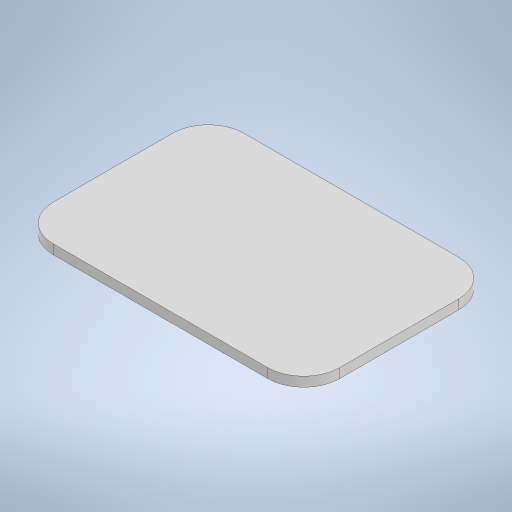
# Autodesk Inventor part: bottom ecoflex layer
Saved by Autodesk Inventor 2024.2 (Build 282272000, 272)
## iProperties
Created: 2025-02-11
Part Number: bottom ecoflex layer
Material: Generic
Document SubType Name: Modeling
Designer: Tom
Density: 1 g/cm^3
Appearance: Default
Author: Tom
Autodesk Inventor part; units mm, degrees
ref_plane "YZ Plane" through (0, 0, 0) normal (1, 0, 0) x (0, 1, 0)
ref_plane "XZ Plane" through (0, 0, 0) normal (0, 1, 0) x (-1, 0, 0)
ref_plane "XY Plane" through (0, 0, 0) normal (0, 0, 1) x (1, 0, 0)
sketch "Sketch1" plane through (0, 0, 0) normal (0, 1, 0) x (-1, 0, 0)
  line L0 (9.525, 0) -> (66.675, 0)
  line L1 (76.2, -9.525) -> (76.2, -41.275)
  line L2 (66.675, -50.8) -> (9.525, -50.8)
  line L3 (0, -41.275) -> (0, -9.525)
  arc A0 (76.2, -9.525) -> (66.675, 0) centre (66.675, -9.525) ccw
  arc A1 (66.675, -50.8) -> (76.2, -41.275) centre (66.675, -41.275) ccw
  arc A2 (0, -41.275) -> (9.525, -50.8) centre (9.525, -41.275) ccw
  arc A3 (9.525, 0) -> (0, -9.525) centre (9.525, -9.525) ccw
  point P0 (0, 0)
  point P1 (76.2, 0)
  point P2 (76.2, -50.8)
  point P3 (0, -50.8)
  dimension "d0" = 50.8
  dimension "d1" = 76.2
  dimension "d2" = 9.525
  dimension "d3" = 9.525
  constraints: 8 end point, 8 point on circle, 8 point on line, 8 tangent, 4 centre point, 3 perpendicular, 2 equal radius, 1 horizontal
  measures "d0" distance of point (76.2, 0) point (76.2, -50.8)
  measures "d1" distance of point (76.2, -50.8) point (0, -50.8)
  measures "d2" radius of A0
  measures "d3" radius of A1
extrude "Extrusion1" add sketch "Sketch1" along normal blind 2.54
body "Solid1"
